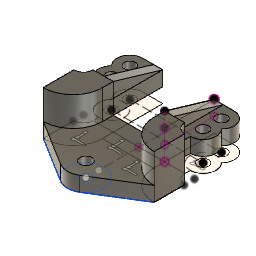
Raspberry Pi Mount v49 (Autodesk Fusion 360 design; units mm, degrees)
Autodesk Fusion 360 part; units mm, degrees
sketch "Sketch1" plane through (0, 0, 0) normal (0, 0, 1) x (1, 0, 0) in component "Component"
  line L0 (7.75, 56) -> (-7.75, 56) construction
  line L1 (-7.75, 56) -> (-7.75, -56) construction
  line L2 (-7.75, -56) -> (7.75, -56) construction
  line L3 (7.75, -56) -> (7.75, 56) construction
  line L4 (7.75, 56) -> (-7.75, -56) construction
  line L5 (-7.75, 56) -> (7.75, -56) construction
  circle A0 centre (-7.75, 56) radius 1.6
  circle A1 centre (7.75, 56) radius 1.6
  circle A2 centre (-7.75, -56) radius 1.6
  circle A3 centre (7.75, -56) radius 1.6
  line L6 (20, 63.5) -> (-20, 63.5)
  line L7 (-20, -63.5) -> (20, -63.5)
  line L8 (20, 63.5) -> (-20, -63.5) construction
  line L9 (-20, 63.5) -> (20, -63.5) construction
  line L10 (15, 50) -> (-15, 50)
  line L11 (-15, 50) -> (-15, -50)
  line L12 (-15, -50) -> (15, -50)
  line L13 (15, -50) -> (15, 50)
  line L14 (15, 50) -> (-15, -50) construction
  line L15 (-15, 50) -> (15, -50) construction
  line L16 (15, -50) -> (20, -50)
  line L17 (-15, -50) -> (-20, -50)
  line L18 (-15, 50) -> (-20, 50)
  line L19 (15, 50) -> (20, 50)
  line L20 (20, -63.5) -> (20, -50)
  line L21 (20, 50) -> (20, 63.5)
  line L22 (-20, 63.5) -> (-20, 50)
  line L23 (-20, -50) -> (-20, -63.5)
  point P0 (0, -63.5)
  dimension "d1_1" = 15.5
  dimension "d2_1" = 112
  dimension "d3_1" = 3.2
  dimension "d4_1" = 3.2
  dimension "d6_1" = 3.2
  dimension "d7_1" = 3.2
  dimension "d8_1" = 40
  dimension "d9_1" = 127
  dimension "d10_1" = 30
  dimension "d11_1" = 100
  constraint perpendicular L0 L1
  constraint parallel L0 L2
  constraint parallel L1 L3
  constraint horizontal L0
  constraint coincident L4 origin
  constraint coincident L5 origin
  constraint coincident L0.end L1.start
  constraint coincident L0.start L3.end
  constraint coincident L1.end L2.start
  constraint coincident L2.end L3.start
  constraint perpendicular L6 L22
  constraint parallel L6 L7
  constraint parallel L20 L22
  constraint horizontal L6
  constraint coincident L8 origin
  constraint coincident L9 origin
  constraint perpendicular L10 L11
  constraint parallel L10 L12
  constraint parallel L11 L13
  constraint horizontal L10
  constraint coincident L14 origin
  constraint coincident L15 origin
  constraint perpendicular L16 L20
  constraint coincident L17.end L22
  constraint perpendicular L17 L22
  constraint perpendicular L18 L22
  constraint coincident L19.end L20
  constraint perpendicular L19 L20
  constraint collinear L20 L21
  constraint collinear L22 L23
  constraint midpoint L7 P0
  measures "d1_1" distance of L1.end L2.end
  measures "d2_1" distance of L0.end L1.end
  measures "d3_1" diameter of A0
  measures "d4_1" diameter of A1
  measures "d6_1" diameter of A2
  measures "d7_1" diameter of A3
  measures "d8_1" distance of L7.start L7.end
  measures "d9_1" distance of L6.end L7.start
  measures "d10_1" distance of L11.end L12.end
  measures "d11_1" distance of L10.end L11.end
extrude "Extrude1" add sketch "Sketch1" along normal blind 5 makes body 1 in component "Component"
sketch "Sketch2" plane through (0, 0, 0) normal (0, 0, 1) x (1, 0, 0) in component "Component"
  circle A0 centre (-7.75, -56) radius 1.6
  circle A1 centre (7.75, -56) radius 1.6
  line L0 (-20, -63.5) -> (20, -63.5)
  line L1 (20, -63.5) -> (20, -52.5)
  line L2 (-20, -63.5) -> (-20, -52.5)
  line L3 (0, -63.5) -> (0, -52.5) construction
  line L4 (-11.875, -52.5) -> (11.875, -52.5) construction
  line L5 (11.875, -52.5) -> (20, -52.5) construction
  line L6 (11.875, -52.5) -> (11.875, -44.5) construction
  line L7 (-11.875, -52.5) -> (-11.875, -44.5) construction
  line L8 (-11.875, -52.5) -> (-20, -52.5) construction
  line L9 (20, -52.5) -> (20, -44.5)
  line L10 (-20, -52.5) -> (-20, -44.5)
  line L11 (-20, -44.5) -> (-11.875, -44.5)
  line L12 (-11.875, -44.5) -> (11.875, -44.5)
  line L13 (11.875, -44.5) -> (20, -44.5)
  arc A2 (-20, -52.5) -> (-11.875, -44.5) centre (-19.876, -44.5) ccw
  arc A3 (11.875, -44.5) -> (20, -52.5) centre (19.876, -44.5) ccw
  dimension "d22_1" = 11
  dimension "d23_1" = 23.75
  dimension "d27_1" = 8
  dimension "d28_1" = 8
  constraint coincident L0.end L1.start
  constraint perpendicular L0 L1
  constraint coincident L0.start L2.start
  constraint perpendicular L0 L2
  constraint midpoint L0 L3.start
  constraint perpendicular L0 L3
  constraint horizontal L4
  constraint midpoint L3.end L4
  constraint perpendicular L1 L5
  constraint perpendicular L2 L8
  constraint perpendicular L5 L9
  constraint perpendicular L8 L10
  constraint perpendicular L7 L11
  constraint perpendicular L6 L12
  constraint perpendicular L9 L13
  constraint collinear L11 L12
  constraint tangent L7 A2
  constraint tangent L6 A3
  measures "d22_1" distance of L3.start L3.end
  measures "d23_1" distance of L4.start L4.end
  measures "d27_1" distance of L1.end L9.end
  measures "d28_1" distance of L2.end L10.end
extrude "Extrude2" add sketch "Sketch2" along normal blind 4 separate body makes body 2 in component "Component"
extrude "Extrude1'" add sketch "Sketch2" along normal blind 12 from surface at 4 separate body contours L10 L11 A2 | L9 L13 A3 makes body 3 at (-15.9473, -51.47, 12) makes body 4 at (12.9677, -48.5362, 12) in component "Joints v47"
sketch "Sketch1 (2)" plane through (0, -44.5, 0) normal (0, 1, 0) x (-1, 0, 0) in component "Joints v47"
  line L0 (-20, 0) -> (20, 0)
  line L1 (20, 0) -> (20, 4)
  line L2 (20, 4) -> (-20, 4)
  line L3 (-20, 4) -> (-20, 0)
  line L4 (11.875, 4) -> (11.875, 16)
  line L5 (20, 4) -> (20, 16)
  line L6 (20, 0) -> (20, 4)
  line L7 (-20, 4) -> (-20, 16)
  line L8 (-20, 0) -> (-20, 4)
  line L9 (-11.875, 4) -> (-11.875, 16)
  line L10 (11.875, 16) -> (20, 16)
  line L11 (-20, 16) -> (-11.875, 16)
  line L12 (-20, 0) -> (20, 0)
  line L13 (11.875, 4) -> (-11.875, 4)
  constraint coincident L4.end L10.start
  constraint coincident L5.end L10.end
  constraint coincident L7.end L11.start
  constraint coincident L9.end L11.end
  constraint coincident L0.start L3.end
  constraint coincident L0.end L1.start
  constraint coincident L4.start L13.start
  constraint coincident L9.start L13.end
extrude "Extrude2'" add sketch "Sketch1 (2)" along normal blind 3 separate body makes body 5 in component "Joints v47"
combine "Combine1" operation add target body 4 tool bodies 5 3 2 in component "Joints v47"
sketch "Sketch1 (3)" plane through (0, 0, 0) normal (0, 0, 1) x (1, 0, 0)
  line L0 (7, -2.9989) -> (7, 0)
  arc A0 (7, -2.9989) -> (15.125, -11) centre (15.125, -2.874) ccw
  circle A1 centre (0, -14.5) radius 1.6
  arc A2 (-15.125, -11) -> (-7, -2.9989) centre (-15.125, -2.874) ccw
  line L1 (-7, -2.9989) -> (-7, 0)
  line L2 (0, 0) -> (0, -11) construction
  line L3 (-15.125, -11) -> (-15.125, -2.625)
  line L4 (-7, 0) -> (-12.5, 0)
  line L5 (-7, 0) -> (7, 0)
  line L6 (7, 0) -> (12.5, 0)
  line L7 (15.125, -2.625) -> (15.125, -11)
  circle A3 centre (0, -14.5) radius 5
  line L8 (15.125, -11) -> (2.6361, -18.7487)
  line L9 (-15.125, -11) -> (-2.6361, -18.7487)
  line L10 (-12.5, 5) -> (12.5, 5) construction
  line L11 (0, 0) -> (0, 5) construction
  line L12 (0, 5) -> (0, 10) construction
  line L13 (-12.5, 10) -> (12.5, 10) construction
  circle A4 centre (12.5, 5) radius 3.5 construction
  line L14 (12.5, 13.5) -> (7, 13.5)
  arc A5 (14.9495, 7.5) -> (12.5, 13.5) centre (12.5, 10) ccw
  arc A6 (12.5, 1.5) -> (14.9495, 7.5) centre (12.5, 5) ccw
  line L15 (12.5, 1.5) -> (12.5, 0)
  line L16 (7, 13.5) -> (7, 0)
  line L17 (-7, 0) -> (-7, 13.5)
  line L18 (-7, 13.5) -> (-12.5, 13.5)
  circle A7 centre (-12.5, 5) radius 3.5 construction
  arc A8 (-12.5, 13.5) -> (-14.9495, 7.5) centre (-12.5, 10) ccw
  arc A9 (-14.9495, 7.5) -> (-12.5, 1.5) centre (-12.5, 5) ccw
  line L19 (-12.5, 1.5) -> (-12.5, 0)
  arc A10 (-15.125, -2.625) -> (-12.5, 0) centre (-15.125, 0) ccw
  arc A11 (12.5, 0) -> (15.125, -2.625) centre (15.125, 0) ccw
  circle A12 centre (-12.5, 5) radius 1.5
  circle A13 centre (-12.5, 10) radius 1.5
  circle A14 centre (12.5, 5) radius 1.5
  circle A15 centre (12.5, 10) radius 1.5
  line L20 (7, -2.9989) -> (-7, -2.9989)
  dimension "d5" = 3.2
  dimension "d35" = 8.125
  dimension "d37" = 8.125
  dimension "d40" = 14
  dimension "d41" = 11
  dimension "d42" = 11
  dimension "d43" = 10
  dimension "d44" = 14.6975
  dimension "d45" = 14.6975
  dimension "d46" = 8.126
  dimension "d47" = 8.0011
  dimension "d50" = 25
  dimension "d51" = 5
  dimension "d52" = 5
  dimension "d53" = 25
  dimension "d57" = 7
  dimension "d58" = 5.5
  dimension "d59" = 3.5
  dimension "d60" = 5.5
  dimension "d61" = 7
  dimension "d62" = 3.5
  dimension "d63" = 2.625
  dimension "d64" = 2.625
  dimension "d65" = 2.625
  dimension "d69" = 3
  dimension "d70" = 3
  dimension "d71" = 3
  dimension "d72" = 3
  constraint coincident L0.end L5.end
  constraint coincident L2.start L11.start
  constraint perpendicular L3 L4
  constraint perpendicular L0 L5
  constraint perpendicular L0 L6
  constraint vertical L7
  constraint symmetric L0 L1 L2
  constraint symmetric L2 L3 L7
  constraint symmetric A0 A2 L2
  constraint midpoint L2.start L5
  constraint coincident A2 L1.start
  constraint coincident L0 A0.start
  constraint coincident L0.start A0
  constraint coincident A2.end L1
  constraint concentric A1 A3
  constraint coincident A3 L8.end
  constraint tangent A3 L8
  constraint coincident A3 L9.end
  constraint tangent A3 L9
  constraint horizontal L4
  constraint horizontal L10
  constraint perpendicular L5 L11
  constraint midpoint L10 L11.end
  constraint perpendicular L10 L12
  constraint perpendicular L12 L13
  constraint midpoint L12.end L13
  constraint coincident L10.end A4.centre
  constraint coincident A4 A5.start
  constraint coincident L13.end A5.centre
  constraint perpendicular L6 L15
  constraint perpendicular L5 L16
  constraint perpendicular L14 L16
  constraint perpendicular L14 L17
  constraint perpendicular L17 L18
  constraint coincident L10.start A7.centre
  constraint coincident A7 A8.end
  constraint coincident L13.start A8.centre
  constraint perpendicular L4 L19
  constraint vertical L15
  constraint concentric A9 A12
  constraint concentric A8 A13
  constraint concentric A6 A14
  constraint concentric A5 A15
  constraint perpendicular L1 L20
  measures "d5" diameter of A1
  measures "d35" distance of L0.end A11.centre
  measures "d37" distance of L1.end A10.centre
  measures "d40" distance of L0.end L1.end
  measures "d41" distance of A2.start A10.centre
  measures "d42" distance of A0.end A11.centre
  measures "d43" diameter of A3
  measures "d44" distance of A2.start L9.end
  measures "d45" distance of A0.end L8.end
  measures "d46" radius of A0
  measures "d47" vertical distance of L0.start A0.end
  measures "d50" distance of L10.start L10.end
  measures "d51" distance of L2.start L11.end
  measures "d52" distance of L11.end L12.end
  measures "d53" distance of L13.start L13.end
  measures "d57" diameter of A4
  measures "d58" distance of L14.start L14.end
  measures "d59" radius of A5
  measures "d60" distance of L17.end L18.end
  measures "d61" diameter of A7
  measures "d62" radius of A8
  measures "d63" radius of A11
  measures "d64" radius of A10
  measures "d65" vertical distance of L6.end L7.start
  measures "d69" diameter of A12
  measures "d70" diameter of A13
  measures "d71" diameter of A14
  measures "d72" diameter of A15
extrude "Extrude1''" add sketch "Sketch1 (3)" along normal blind 4 separate body contours L0 L1 L5 L20 | A0 A2 A3 L8 L9 L20 | A3 makes body 6
extrude "Extrude2''" add sketch "Sketch1 (3)" along normal blind 12 separate body contours L0 A0 L6 L7 A11 | A2 L1 L3 L4 A10 makes body 7 at (10.1436, -9.2941, 8) makes body 8 at (-7.0149, -3.3816, 8)
extrude "Extrude9" add sketch "Sketch1 (3)" along normal blind 4 from surface at 4 separate body contours L6 L14 A5 A6 L15 L16 | L4 L17 L18 A8 A9 L19 makes body 9 at (-8.3389, 6.2412, 4) makes body 10 at (8.3389, 6.2412, 4)
sketch "Sketch4" plane through (7, 0, 0) normal (-1, 0, 0) x (0, -1, 0)
  line L0 (-13.5, 4) -> (0, 4)
  line L1 (0, 4) -> (0, 8)
  line L2 (0, 8) -> (-13.5, 8)
  line L3 (-13.5, 8) -> (-13.5, 4)
  line L4 (-13.5, 4) -> (-13.5, 8)
  line L5 (0, 4) -> (0, 8)
  line L6 (0, 4) -> (-13.5, 4)
  line L7 (0, 0) -> (0, 12)
  line L8 (0, 12) -> (-13.5, 8)
  line L9 (0, 8) -> (-13.5, 8)
  constraint coincident L7.end L8.start
  constraint coincident L2.end L3.start
  constraint coincident L1.end L2.start
extrude "Extrude12" add sketch "Sketch4" against normal blind 2.5 contours L2 L7 L8 L9 bodies 7 10
extrude "Extrude13" add sketch "Sketch4" along normal blind 2.5 from surface at 14 separate body contours L2 L7 L8 L9 makes body 11
component "Joints v47" placed x (1, 0, 0) y (0, 1, 0) z (0, 0, 1) at (0, 41.5, 0)
component "Component" placed x (1, 0, 0) y (0, 1, 0) z (0, 0, 1) at (0, 0, 0) in component "Joints v47"
hidden bodies 1
equation "d4_1 = radius"
equation "radius = 3.2 mm"
equation "d6_1 = radius"
equation "d7_1 = radius"
